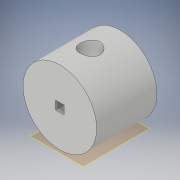
# Autodesk Inventor part: powderTurn
Saved by Autodesk Inventor 2017 (Build 210142000, 142)
## iProperties
Created: 2019-05-09
Part Number: powderTurn
Material: Generic
Document SubType Name: Modeling
Designer: Joe Sedutto
Density: 1 g/cm^3
Appearance: Default
Author: Joe Sedutto
Autodesk Inventor part; units mm, degrees
ref_plane "YZ Plane" through (0, 0, 0) normal (1, 0, 0) x (0, 1, 0)
ref_plane "XY Plane" through (0, 0, 0) normal (0, 0, 1) x (1, 0, 0)
sketch "Sketch1" plane through (0, 0, 0) normal (0, 0, 1) x (1, 0, 0)
  circle A0 centre (0, 0) radius 15.494
  dimension "d0" = 30.988
  constraints: 1 centre point, 1 coincident
  measures "d0" diameter of A0
extrude "Extrusion1" add sketch "Sketch1" along normal blind 25.4
ref_plane "Work Plane2" through (0, 15.494, 0) normal (0, 1, 0) x (-1, 0, 0)
ref_plane "Work Plane1" through (0, -15.494, 0) normal (0, 1, 0) x (-1, 0, 0)
sketch "Sketch2" plane through (0, 15.494, 0) normal (0, 1, 0) x (-1, 0, 0)
  point P0 (0, 0)
  point P1 (0, 12.7)
  dimension "d3" = 12.7
  dimension "d4" = 0
  measures "d3" distance of point (0, 0) point (0, 12.7)
  measures "d4" horizontal distance of point (0, 12.7) point (0, 0)
sketch "Sketch3" plane through (0, -15.494, 0) normal (0, 1, 0) x (-1, 0, 0)
  point P0 (0, 0)
  point P1 (0, 12.7)
  dimension "d5" = 12.7
  dimension "d6" = 0
  measures "d5" distance of point (0, 0) point (0, 12.7)
  measures "d6" horizontal distance of point (0, 0) point (0, 12.7)
hole "Hole1" at (0, 15.494, 12.7) direction (0, -1, 0) diameter 8.382 depth 6.35 tip angle 60
hole "Hole2" at (0, -15.494, 12.7) direction (0, 1, 0) diameter 8.382 depth 6.35 tip angle 60
sketch "Sketch4" plane through (0, 0, 25.4) normal (0, 0, 1) x (1, 0, 0)
  line L0 (-1.778, -1.778) -> (1.778, -1.778)
  line L1 (1.778, -1.778) -> (1.778, 1.778)
  line L2 (1.778, 1.778) -> (-1.778, 1.778)
  line L3 (-1.778, 1.778) -> (-1.778, -1.778)
  line L4 (-1.778, -1.778) -> (1.778, 1.778) construction
  line L5 (1.778, -1.778) -> (-1.778, 1.778) construction
  point P0 (0, 0)
  dimension "d21" = 3.556
  dimension "d22" = 3.556
  constraints: 12 end point, 2 midpoint, 2 parallel, 1 horizontal, 1 perpendicular
  measures "d21" distance of L2.end L1.end
  measures "d22" distance of L1.end L0.end
extrude "Extrusion2" cut sketch "Sketch4" against normal blind 25.4
body "Solid1"
